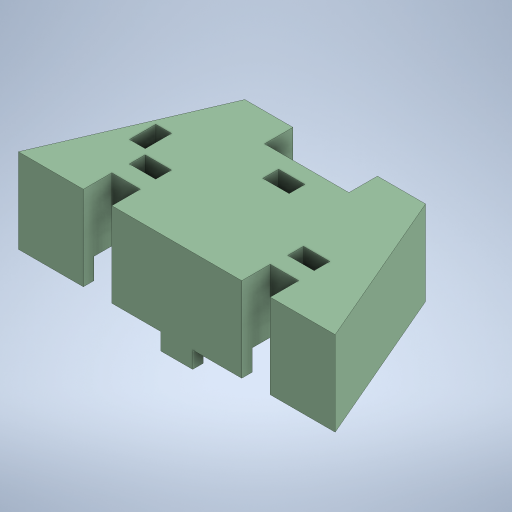
# Autodesk Inventor part: MUX
Saved by Autodesk Inventor 2024.3 (Build 283343000, 343)
## iProperties
Created: 2024-03-15
Part Number: MUX
Material: Generic
Document SubType Name: Modeling
Designer: Jonat
Density: 1 g/cm^3
Appearance: Rubber - Green
Author: Jonat
Autodesk Inventor part; units mm, degrees
ref_plane "YZ Plane" through (0, 0, 0) normal (1, 0, 0) x (0, 1, 0)
ref_plane "XZ Plane" through (0, 0, 0) normal (0, 1, 0) x (-1, 0, 0)
ref_plane "XY Plane" through (0, 0, 0) normal (0, 0, 1) x (1, 0, 0)
sketch "Sketch1" plane through (0, 0, 0) normal (0, 1, 0) x (-1, 0, 0)
  line L0 (-15, 7.5) -> (15, 7.5)
  line L1 (15, 7.5) -> (15, -7.5)
  line L2 (15, -7.5) -> (-15, -7.5)
  line L3 (-15, -7.5) -> (-15, 7.5)
  line L4 (-15, 7.5) -> (15, -7.5) construction
  line L5 (15, 7.5) -> (-15, -7.5) construction
  point P0 (0, 0)
  dimension "d0" = 30
  dimension "d1" = 15
  constraints: 12 end point, 2 midpoint, 2 parallel, 1 horizontal, 1 perpendicular
  measures "d0" distance of L1.end L2.end
  measures "d1" distance of L0.end L1.end
extrude "Extrusion1" add sketch "Sketch1" along normal blind 8
sketch "Sketch3" plane through (0, 8, 0) normal (0, 1, 0) x (1, 0, 0)
  line L0 (-15, 7.5) -> (-15, -7.5) projected
  line L1 (-15, -7.5) -> (15, -7.5) projected
  line L2 (-15, -7.5) -> (15, -7.5)
  line L3 (15, -7.5) -> (8.5, 7.6369)
  line L4 (-15, -7.5) -> (-8.5, 7.6369)
  line L5 (-8.5, 7.6369) -> (8.5, 7.6369)
  line L6 (-10.75, -1.2417) -> (-9.25, -1.2417)
  line L7 (-9.25, -1.2417) -> (-9.25, 1.2583)
  line L8 (-9.25, 1.2583) -> (-10.75, 1.2583)
  line L9 (-10.75, 1.2583) -> (-10.75, -1.2417)
  line L10 (-10.75, -1.2417) -> (-9.25, 1.2583) construction
  line L11 (-9.25, -1.2417) -> (-10.75, 1.2583) construction
  line L12 (-6.25, -3.25) -> (-8.75, -3.25)
  line L13 (-8.75, -3.25) -> (-8.75, -1.75)
  line L14 (-8.75, -1.75) -> (-6.25, -1.75)
  line L15 (-6.25, -1.75) -> (-6.25, -3.25)
  line L16 (-6.25, -3.25) -> (-8.75, -1.75) construction
  line L17 (-8.75, -3.25) -> (-6.25, -1.75) construction
  line L18 (8.75, -1.75) -> (6.25, -1.75)
  line L19 (6.25, -1.75) -> (6.25, -3.25)
  line L20 (6.25, -3.25) -> (8.75, -3.25)
  line L21 (8.75, -3.25) -> (8.75, -1.75)
  line L22 (8.75, -1.75) -> (6.25, -3.25) construction
  line L23 (6.25, -1.75) -> (8.75, -3.25) construction
  line L24 (15, 7.5) -> (-15, 7.5) projected
  line L25 (-15, -7.5) -> (-15, 7.5)
  line L26 (-15, 7.5) -> (15, 7.5)
  line L27 (15, 7.5) -> (15, -7.5)
  line L28 (1.25, 1.8869) -> (-1.25, 1.8869)
  line L29 (-1.25, 1.8869) -> (-1.25, 3.3869)
  line L30 (-1.25, 3.3869) -> (1.25, 3.3869)
  line L31 (1.25, 3.3869) -> (1.25, 1.8869)
  line L32 (1.25, 1.8869) -> (-1.25, 3.3869) construction
  line L33 (-1.25, 1.8869) -> (1.25, 3.3869) construction
  point P0 (0, 0)
  point P1 (-10, 0.0083)
  point P2 (-7.5, -2.5)
  point P3 (7.5, -2.5)
  point P4 (0, -7.5)
  point P5 (0, -7.5)
  point P6 (0, 2.6369)
  point P7 (8.5588, 7.5)
  point P8 (-8.5588, 7.5)
  dimension "d19" = 17
  dimension "d20" = 1.5
  dimension "d21" = 2.5
  dimension "d22" = 5
  dimension "d24" = 7.5
  dimension "d25" = 7.5
  dimension "d26" = 5
  dimension "d27" = 5
  dimension "d28" = 5
  dimension "d29" = 0
  constraints: 62 end point, 10 midpoint, 9 parallel, 7 equal length, 5 horizontal, 5 perpendicular, 1 collinear, 1 vertical
  measures "d19" distance of L4.end L3.end
  measures "d20" distance of L8.end L7.end
  measures "d21" distance of L7.end L6.end
  measures "d22" distance from line of L0 point (-10, 0.008)
  measures "d24" horizontal distance of point (0, -7.5) point (-7.5, -2.5)
  measures "d25" horizontal distance of point (0, -7.5) point (7.5, -2.5)
  measures "d26" distance from line of L1 point (-7.5, -2.5)
  measures "d27" distance from line of L1 point (7.5, -2.5)
  measures "d28" distance from line of point (0, 2.637) L5
  measures "d29" horizontal distance of point (0, 0) point (0, 2.637)
extrude "Extrusion3" cut sketch "Sketch3" against normal blind 8 contours L24 L4 L0 | L3 L24 L27 | L9 L8 L7 L6 | L12 L13 L14 L15 | L21 L20 L19 L18 | L28 L29 L30 L31
sketch "Sketch4" plane through (0, 0, 0) normal (0, -1, 0) x (1, 0, 0)
  line L0 (-9.25, 1.7417) -> (-10.75, 1.7417)
  line L1 (-10.75, 1.7417) -> (-10.75, -1.7583)
  line L2 (-10.75, -1.7583) -> (-9.25, -1.7583)
  line L3 (-9.25, -1.7583) -> (-9.25, 1.7417)
  line L4 (-9.25, 1.7417) -> (-10.75, -1.7583) construction
  line L5 (-10.75, 1.7417) -> (-9.25, -1.7583) construction
  line L6 (-10.75, -1.2583) -> (-10.75, 1.2417) projected
  line L7 (-9.25, 1.2417) -> (-9.25, -1.2583) projected
  line L8 (-9.25, -1.2583) -> (-10.75, -1.2583) projected
  line L9 (-10.75, 1.2417) -> (-9.25, 1.2417) projected
  line L10 (-8.75, 3.25) -> (-6.25, 3.25) construction
  line L11 (-7.5, 3.25) -> (-7.5, 1.75) construction
  line L12 (-8.75, 1.75) -> (-6.25, 1.75) construction
  line L13 (-1.25, -1.8869) -> (1.25, -1.8869) construction
  line L14 (0, -1.8869) -> (0, -3.3869) construction
  line L15 (1.25, -3.3869) -> (-1.25, -3.3869) construction
  line L16 (6.25, 3.25) -> (8.75, 3.25) construction
  line L17 (7.5, 3.25) -> (7.5, 1.75) construction
  line L18 (8.75, 1.75) -> (6.25, 1.75) construction
  line L19 (9.25, 3.25) -> (5.75, 3.25)
  line L20 (5.75, 3.25) -> (5.75, 1.75)
  line L21 (5.75, 1.75) -> (9.25, 1.75)
  line L22 (9.25, 1.75) -> (9.25, 3.25)
  line L23 (9.25, 3.25) -> (5.75, 1.75) construction
  line L24 (5.75, 3.25) -> (9.25, 1.75) construction
  line L25 (1.75, -1.8869) -> (-1.75, -1.8869)
  line L26 (-1.75, -1.8869) -> (-1.75, -3.3869)
  line L27 (-1.75, -3.3869) -> (1.75, -3.3869)
  line L28 (1.75, -3.3869) -> (1.75, -1.8869)
  line L29 (1.75, -1.8869) -> (-1.75, -3.3869) construction
  line L30 (-1.75, -1.8869) -> (1.75, -3.3869) construction
  line L31 (-5.75, 3.25) -> (-9.25, 3.25)
  line L32 (-9.25, 3.25) -> (-9.25, 1.75)
  line L33 (-9.25, 1.75) -> (-5.75, 1.75)
  line L34 (-5.75, 1.75) -> (-5.75, 3.25)
  line L35 (-5.75, 3.25) -> (-9.25, 1.75) construction
  line L36 (-9.25, 3.25) -> (-5.75, 1.75) construction
  point P0 (0, 0)
  point P1 (-10, -0.0083)
  point P2 (7.5, 2.5)
  point P3 (0, -2.6369)
  point P4 (-7.5, 2.5)
  point P5 (-10.75, 1.2417)
  dimension "d32" = 0
  dimension "d33" = 0
  dimension "d34" = 0.5
  dimension "d35" = 0.5
  dimension "d36" = 3.5
  dimension "d37" = 3.5
  dimension "d38" = 3.5
  constraints: 54 end point, 17 midpoint, 8 parallel, 5 perpendicular, 4 horizontal
  measures "d32" distance between parallel lines of L6 L1
  measures "d33" distance between parallel lines of L7 L3
  measures "d34" distance between parallel lines of L8 L2
  measures "d35" distance between parallel lines of L0 L9
  measures "d36" distance of L21.end L20.end
  measures "d37" distance of L27.end L26.end
  measures "d38" distance of L33.end L32.end
extrude "Extrusion4" cut sketch "Sketch4" against normal blind 3.5
sketch "Sketch5" plane through (0, 0, 0) normal (0, -1, 0) x (1, 0, 0)
  line L0 (-9.25, -1.7583) -> (-10.75, -1.7583) projected
  line L1 (-15, 7.5) -> (-8.5588, -7.5) projected
  line L2 (8.5588, -7.5) -> (-8.5588, -7.5) projected
  line L3 (-7.8999, -6.5) -> (7.8999, -6.5)
  line L4 (7.8999, -6.5) -> (13.4823, 6.5)
  line L5 (8.5588, -7.5) -> (15, 7.5) projected
  line L6 (-15, 7.5) -> (15, 7.5) projected
  line L7 (13.4823, 6.5) -> (-14, 6.5)
  line L8 (-7.8999, -6.5) -> (-13.4823, 6.5)
  point P0 (0, 0)
  point P1 (-13.4823, 6.5)
  dimension "d41" = 1
  dimension "d42" = 1
  dimension "d43" = 1
  dimension "d44" = 1
  dimension "d45" = 1
  dimension "d46" = 1
  constraints: 8 end point, 2 horizontal, 2 parallel
  measures "d41" distance from line of L2 L3.start
  measures "d42" distance between parallel lines of L5 L4
  measures "d43" distance from line of L6 L4.end
  measures "d44" distance between parallel lines of L1 L8
  measures "d45" distance from line of L6 L8.end
  measures "d46" horizontal distance of L1.start L7.end
sketch "Sketch2" plane through (0, 8, 0) normal (0, 1, 0) x (1, 0, 0)
  line L0 (4, 7.5) -> (-4, 7.5)
  line L1 (-4, 7.5) -> (-4, 4.8)
  line L2 (-4, 4.8) -> (4, 4.8)
  line L3 (4, 4.8) -> (4, 7.5)
  line L4 (4, 7.5) -> (-4, 4.8) construction
  line L5 (-4, 7.5) -> (4, 4.8) construction
  line L6 (-6.15, -4.8) -> (-8.85, -4.8)
  line L7 (-8.85, -4.8) -> (-8.85, -7.5)
  line L8 (-8.85, -7.5) -> (-6.15, -7.5)
  line L9 (-6.15, -7.5) -> (-6.15, -4.8)
  line L10 (-6.15, -4.8) -> (-8.85, -7.5) construction
  line L11 (-8.85, -4.8) -> (-6.15, -7.5) construction
  line L12 (8.85, -4.8) -> (6.15, -4.8)
  line L13 (6.15, -4.8) -> (6.15, -7.5)
  line L14 (6.15, -7.5) -> (8.85, -7.5)
  line L15 (8.85, -7.5) -> (8.85, -4.8)
  line L16 (8.85, -4.8) -> (6.15, -7.5) construction
  line L17 (6.15, -4.8) -> (8.85, -7.5) construction
  point P0 (0, 0)
  point P1 (0, 6.15)
  point P2 (-7.5, -6.15)
  point P3 (7.5, -6.15)
  dimension "d8" = 8
  dimension "d9" = 2.7
  dimension "d10" = 7.5
  dimension "d11" = 2.7
  dimension "d12" = 7.5
  dimension "d13" = 7.5
  dimension "d15" = 7.5
  dimension "d16" = 7.5
  constraints: 36 end point, 6 midpoint, 6 parallel, 6 perpendicular, 3 horizontal
  measures "d8" distance of L2.end L1.end
  measures "d9" distance of L1.end L0.end
  measures "d10" distance from line of point (0, 0) L0
  measures "d11" distance of L8.end L7.end
  measures "d12" horizontal distance of point (0, 0) point (7.5, -6.15)
  measures "d13" distance from line of point (0, 0) L14
  measures "d15" distance from line of point (0, 0) L8
  measures "d16" horizontal distance of point (0, 0) point (-7.5, -6.15)
extrude "Extrusion2" cut sketch "Sketch2" against normal blind 8
extrude "Extrusion5" cut sketch "Sketch5" against normal blind 2 contours L8 L7 L4 L3
sketch "Sketch6" plane through (0, 2, 0) normal (0, -1, 0) x (1, 0, 0)
  circle A0 centre (0, 0) radius 1
  circle A1 centre (0, 0) radius 1.6
  dimension "d49" = 2
  dimension "d50" = 0.6
  constraints: 2 centre point, 2 coincident
  measures "d49" diameter of A0
  measures "d50" radial gap between concentric circles of A0 A1
extrude "Extrusion6" add sketch "Sketch6" along normal blind 2
sketch "Sketch7" plane through (0, 0, 0) normal (0, -1, 0) x (1, 0, 0)
  circle A0 centre (0, 0) radius 1
  dimension "d74" = 2
  constraints: 1 centre point, 1 coincident
  measures "d74" diameter of A0
extrude "Extrusion7" cut sketch "Sketch7" against normal blind 5
sketch "Sketch8" plane through (0, 0, 0) normal (0, -1, 0) x (1, 0, 0)
  line L0 (-7.5, -7.5) -> (-4.5, -7.5)
  line L1 (-4.5, -7.5) -> (-4.5, -6.5)
  line L2 (-4.5, -6.5) -> (-7.5, -6.5)
  line L3 (-7.5, -6.5) -> (-7.5, -7.5)
  line L4 (7.5, -6.5) -> (5, -6.5)
  line L5 (5, -6.5) -> (5, -7.5)
  line L6 (5, -7.5) -> (7.5, -7.5)
  line L7 (7.5, -7.5) -> (7.5, -6.5)
  line L8 (1.5, 7.5) -> (-1.5, 7.5)
  line L9 (-1.5, 7.5) -> (-1.5, 6.5)
  line L10 (-1.5, 6.5) -> (1.5, 6.5)
  line L11 (1.5, 6.5) -> (1.5, 7.5)
  line L12 (1.5, 7.5) -> (-1.5, 6.5) construction
  line L13 (-1.5, 7.5) -> (1.5, 6.5) construction
  point P0 (0, 0)
  point P1 (0, 7)
  point P2 (-6, -6.5)
  point P3 (6.25, -7.5)
  point P4 (-6, -7.5)
  dimension "d55" = 3
  dimension "d56" = 1
  dimension "d57" = 2.5
  dimension "d58" = 1
  dimension "d59" = 3
  dimension "d60" = 1
  dimension "d62" = 7.5
  dimension "d63" = 7.5
  dimension "d64" = 7.5
  dimension "d72" = 9.5
  dimension "d73" = 6
  constraints: 28 end point, 6 parallel, 5 midpoint, 3 horizontal, 3 perpendicular, 1 point on line
  measures "d55" distance of L2.end L1.end
  measures "d56" distance of L1.end L0.end
  measures "d57" distance of L6.end L5.end
  measures "d58" distance of L5.end L4.end
  measures "d59" distance of L10.end L9.end
  measures "d60" distance of L9.end L8.end
  measures "d62" distance from line of point (0, 0) L8
  measures "d63" distance from line of point (0, 0) L6
  measures "d64" distance from line of point (0, 0) L0
  measures "d72" distance between parallel lines of L5 L1
  measures "d73" horizontal distance of point (-6, -7.5) point (0, 0)
extrude "Extrusion8" add sketch "Sketch8" along normal blind 1.6
body "Solid1"
